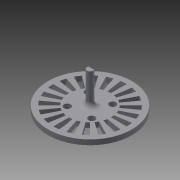
# Autodesk Inventor part: EncoderWheelAndPotInsert2
Saved by Autodesk Inventor 2014 SP2 (Build 180246200, 246)
## iProperties
Created: 2014-11-03
Part Number: EncoderWheelAndPotInsert2
Material: Generic
Document SubType Name: Modeling
Designer: Rebecca
Density: 1 g/cm^3
Appearance: Default
Author: Rebecca
Autodesk Inventor part; units mm, degrees
ref_plane "YZ Plane" through (0, 0, 0) normal (1, 0, 0) x (0, 1, 0)
ref_plane "XZ Plane" through (0, 0, 0) normal (0, 1, 0) x (-1, 0, 0)
ref_plane "XY Plane" through (0, 0, 0) normal (0, 0, 1) x (1, 0, 0)
sketch "Sketch1" plane through (0, 0, 0) normal (0, 1, 0) x (-1, 0, 0)
  circle A0 centre (0, 0) radius 25.4
  arc A1 (22.225, 0) -> (21.9514, 3.4768) centre (0, 0) ccw
  arc A2 (12.7, 0) -> (12.5436, 1.9867) centre (0, 0) ccw
  line L0 (12.7, 0) -> (22.225, 0)
  line L1 (12.5436, 1.9867) -> (21.9514, 3.4768)
  line L2 (12.7, 0) -> (22.225, 0) construction
  arc A3 (21.1372, -6.8679) -> (21.9514, -3.4768) centre (0, 0) ccw
  arc A4 (12.0784, -3.9245) -> (12.5436, -1.9867) centre (0, 0) ccw
  line L3 (12.0784, -3.9245) -> (21.1372, -6.8679)
  line L4 (12.5436, -1.9867) -> (21.9514, -3.4768)
  arc A5 (17.9804, -13.0635) -> (19.8026, -10.0899) centre (0, 0) ccw
  arc A6 (10.2745, -7.4649) -> (11.3158, -5.7657) centre (0, 0) ccw
  line L5 (10.2745, -7.4649) -> (17.9804, -13.0635)
  line L6 (11.3158, -5.7657) -> (19.8026, -10.0899)
  arc A7 (13.0635, -17.9804) -> (15.7154, -15.7154) centre (0, 0) ccw
  arc A8 (7.4649, -10.2745) -> (8.9803, -8.9803) centre (0, 0) ccw
  line L7 (7.4649, -10.2745) -> (13.0635, -17.9804)
  line L8 (8.9803, -8.9803) -> (15.7154, -15.7154)
  arc A9 (6.8679, -21.1372) -> (10.0899, -19.8026) centre (0, 0) ccw
  arc A10 (3.9245, -12.0784) -> (5.7657, -11.3158) centre (0, 0) ccw
  line L9 (3.9245, -12.0784) -> (6.8679, -21.1372)
  line L10 (5.7657, -11.3158) -> (10.0899, -19.8026)
  arc A11 (0, -22.225) -> (3.4768, -21.9514) centre (0, 0) ccw
  arc A12 (0, -12.7) -> (1.9867, -12.5436) centre (0, 0) ccw
  line L11 (0, -12.7) -> (0, -22.225)
  line L12 (1.9867, -12.5436) -> (3.4768, -21.9514)
  arc A13 (-6.8679, -21.1372) -> (-3.4768, -21.9514) centre (0, 0) ccw
  arc A14 (-3.9245, -12.0784) -> (-1.9867, -12.5436) centre (0, 0) ccw
  line L13 (-3.9245, -12.0784) -> (-6.8679, -21.1372)
  line L14 (-1.9867, -12.5436) -> (-3.4768, -21.9514)
  arc A15 (-13.0635, -17.9804) -> (-10.0899, -19.8026) centre (0, 0) ccw
  arc A16 (-7.4649, -10.2745) -> (-5.7657, -11.3158) centre (0, 0) ccw
  line L15 (-7.4649, -10.2745) -> (-13.0635, -17.9804)
  line L16 (-5.7657, -11.3158) -> (-10.0899, -19.8026)
  arc A17 (-17.9804, -13.0635) -> (-15.7154, -15.7154) centre (0, 0) ccw
  arc A18 (-10.2745, -7.4649) -> (-8.9803, -8.9803) centre (0, 0) ccw
  line L17 (-10.2745, -7.4649) -> (-17.9804, -13.0635)
  line L18 (-8.9803, -8.9803) -> (-15.7154, -15.7154)
  arc A19 (-21.1372, -6.8679) -> (-19.8026, -10.0899) centre (0, 0) ccw
  arc A20 (-12.0784, -3.9245) -> (-11.3158, -5.7657) centre (0, 0) ccw
  line L19 (-12.0784, -3.9245) -> (-21.1372, -6.8679)
  line L20 (-11.3158, -5.7657) -> (-19.8026, -10.0899)
  arc A21 (-22.225, 0) -> (-21.9514, -3.4768) centre (0, 0) ccw
  arc A22 (-12.7, 0) -> (-12.5436, -1.9867) centre (0, 0) ccw
  line L21 (-12.7, 0) -> (-22.225, 0)
  line L22 (-12.5436, -1.9867) -> (-21.9514, -3.4768)
  arc A23 (-21.1372, 6.8679) -> (-21.9514, 3.4768) centre (0, 0) ccw
  arc A24 (-12.0784, 3.9245) -> (-12.5436, 1.9867) centre (0, 0) ccw
  line L23 (-12.0784, 3.9245) -> (-21.1372, 6.8679)
  line L24 (-12.5436, 1.9867) -> (-21.9514, 3.4768)
  arc A25 (-17.9804, 13.0635) -> (-19.8026, 10.0899) centre (0, 0) ccw
  arc A26 (-10.2745, 7.4649) -> (-11.3158, 5.7657) centre (0, 0) ccw
  line L25 (-10.2745, 7.4649) -> (-17.9804, 13.0635)
  line L26 (-11.3158, 5.7657) -> (-19.8026, 10.0899)
  arc A27 (-13.0635, 17.9804) -> (-15.7154, 15.7154) centre (0, 0) ccw
  arc A28 (-7.4649, 10.2745) -> (-8.9803, 8.9803) centre (0, 0) ccw
  line L27 (-7.4649, 10.2745) -> (-13.0635, 17.9804)
  line L28 (-8.9803, 8.9803) -> (-15.7154, 15.7154)
  arc A29 (-6.8679, 21.1372) -> (-10.0899, 19.8026) centre (0, 0) ccw
  arc A30 (-3.9245, 12.0784) -> (-5.7657, 11.3158) centre (0, 0) ccw
  line L29 (-3.9245, 12.0784) -> (-6.8679, 21.1372)
  line L30 (-5.7657, 11.3158) -> (-10.0899, 19.8026)
  arc A31 (0, 22.225) -> (-3.4768, 21.9514) centre (0, 0) ccw
  arc A32 (0, 12.7) -> (-1.9867, 12.5436) centre (0, 0) ccw
  line L31 (0, 12.7) -> (0, 22.225)
  line L32 (-1.9867, 12.5436) -> (-3.4768, 21.9514)
  arc A33 (6.8679, 21.1372) -> (3.4768, 21.9514) centre (0, 0) ccw
  arc A34 (3.9245, 12.0784) -> (1.9867, 12.5436) centre (0, 0) ccw
  line L33 (3.9245, 12.0784) -> (6.8679, 21.1372)
  line L34 (1.9867, 12.5436) -> (3.4768, 21.9514)
  arc A35 (13.0635, 17.9804) -> (10.0899, 19.8026) centre (0, 0) ccw
  arc A36 (7.4649, 10.2745) -> (5.7657, 11.3158) centre (0, 0) ccw
  line L35 (7.4649, 10.2745) -> (13.0635, 17.9804)
  line L36 (5.7657, 11.3158) -> (10.0899, 19.8026)
  arc A37 (17.9804, 13.0635) -> (15.7154, 15.7154) centre (0, 0) ccw
  arc A38 (10.2745, 7.4649) -> (8.9803, 8.9803) centre (0, 0) ccw
  line L37 (10.2745, 7.4649) -> (17.9804, 13.0635)
  line L38 (8.9803, 8.9803) -> (15.7154, 15.7154)
  arc A39 (21.1372, 6.8679) -> (19.8026, 10.0899) centre (0, 0) ccw
  arc A40 (12.0784, 3.9245) -> (11.3158, 5.7657) centre (0, 0) ccw
  line L39 (12.0784, 3.9245) -> (21.1372, 6.8679)
  line L40 (11.3158, 5.7657) -> (19.8026, 10.0899)
  line L41 (-6.3513, -7.4364) -> (6.3513, 7.4364) construction
  line L42 (7.4364, -6.3513) -> (-7.4364, 6.3513) construction
  circle A41 centre (-7.4364, 6.3513) radius 2.032
  circle A42 centre (6.3513, 7.4364) radius 2.032
  circle A43 centre (7.4364, -6.3513) radius 2.032
  circle A44 centre (-6.3513, -7.4364) radius 2.032
  dimension "d0" = 50.8
  dimension "d3" = 9
  dimension "d6" = 360
  dimension "d8" = 13.8303
  dimension "d9" = 13.8303
  dimension "d10" = 4.064
  dimension "d11" = 4.064
  dimension "d12" = 4.064
  dimension "d13" = 4.064
  constraints: 86 end point, 80 point on circle, 45 centre point, 27 coincident, 2 horizontal, 2 midpoint, 218 other
  measures "d0" diameter of A0
  measures "d3" angle of L2 L1
  measures "d8" distance of L42.end L41.end
  measures "d9" distance of L41.end L42.start
  measures "d10" diameter of A41
  measures "d11" diameter of A42
  measures "d12" diameter of A43
  measures "d13" diameter of A44
extrude "Extrusion1" add sketch "Sketch1" along normal blind 3.048
sketch "Sketch2" plane through (0, 3.048, 0) normal (0, 1, 0) x (1, 0, 0)
  circle A0 centre (0, 0) radius 25.4 projected
  arc A1 (-1.6848, 0.889) -> (1.6848, 0.889) centre (0, 0) ccw
  line L0 (1.6848, 0.889) -> (-1.6848, 0.889)
  dimension "d16" = 3.81
  constraints: 2 end point, 2 point on circle, 1 centre point, 1 coincident
  measures "d16" diameter of A1
extrude "Extrusion2" add sketch "Sketch2" along normal blind 19.05 contours L0 A1
fillet "Fillet1" radius 3.175 2 edges at (0, 3.048, 1.905) (0, 3.048, -0.889)
body "Solid1"
